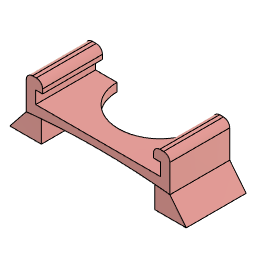
MPR121_Clip (Autodesk Fusion 360 design; units mm, degrees)
Autodesk Fusion 360 part; units mm, degrees
note: some values were not read from the file. Set by a fixed rule: which sketch regions a step uses.
sketch "Clip Sketch" plane through (0, 0, 0) normal (0, 0, 1) x (1, 0, 0)
  line L0 (9.9, 4.75) -> (-9.9, 4.75)
  line L1 (-9.9, 4.75) -> (-9.9, -4.75)
  line L2 (-9.9, -4.75) -> (9.9, -4.75)
  line L3 (9.9, -4.75) -> (9.9, 4.75)
  line L4 (9.9, 4.75) -> (-9.9, -4.75) construction
  line L5 (-9.9, 4.75) -> (9.9, -4.75) construction
  line L6 (-9.9, 4.75) -> (-11.4, 4.75)
  line L7 (-11.4, 4.75) -> (-11.4, -4.75)
  line L8 (-11.4, -4.75) -> (-9.9, -4.75)
  line L9 (-9.9, -4.75) -> (-9.9, 4.75)
  line L10 (9.9, -4.75) -> (11.4, -4.75)
  line L11 (11.4, -4.75) -> (11.4, 4.75)
  line L12 (11.4, 4.75) -> (9.9, 4.75)
  line L13 (9.9, 4.75) -> (9.9, -4.75)
  line L14 (-9.9, -4.75) -> (-8.8, -4.75)
  line L15 (-8.8, -4.75) -> (-8.8, 4.75)
  line L16 (-8.8, 4.75) -> (-9.9, 4.75)
  line L17 (-9.9, 4.75) -> (-9.9, -4.75)
  line L18 (0, 2.5) -> (0, 20)
  line L19 (8.8, -4.75) -> (8.8, 4.75)
  line L20 (9.9, -4.75) -> (8.8, -4.75)
  line L21 (8.8, 4.75) -> (9.9, 4.75)
  line L22 (-11.4, 4.75) -> (-11.4, 0.75)
  dimension "d1" = 19.8
  dimension "d2" = 9.5
  dimension "d3" = 1.5
  dimension "d4" = 1.5
  dimension "d5" = 1.1
  dimension "d18" = 4
  constraint horizontal L0
  constraint perpendicular L0 L1
  constraint parallel L0 L2
  constraint parallel L1 L3
  constraint coincident L4 origin
  constraint coincident L5 origin
  constraint horizontal L6
  constraint vertical L7
  constraint horizontal L8
  constraint vertical L9
  constraint horizontal L10
  constraint vertical L11
  constraint horizontal L12
  constraint vertical L13
  constraint collinear L0 L12
  constraint collinear L2 L8
  constraint horizontal L14
  constraint vertical L15
  constraint horizontal L16
  constraint vertical L17
  constraint coincident L9 L1.end
  constraint symmetric L1.end L18 L2.end
  constraint symmetric L14.end L18 L19.start
  constraint symmetric L15.end L18 L19.end
  constraint symmetric L0.end L18 L0.start
  constraint vertical L22
  constraint coincident L7 L22.end
  constraint collinear L0 L16
  constraint collinear L2 L14
  measures "d1" distance of L1.end L2.end
  measures "d2" distance of L0.end L1.end
  measures "d3" distance of L0.end L6.end
  measures "d4" distance of L2.end L10.end
  measures "d5" distance of L1.end L14.end
  measures "d18" distance of L22.end L6.end
extrude "Extrude1" add sketch "Clip Sketch" along normal blind 2
extrude "Extrude2" add sketch "Clip Sketch" along normal blind 4 contours L3 L10 L11 L12 L13 | L1 L6 L7 L8 L9 L17 L22
extrude "Extrude3" add sketch "Clip Sketch" along normal blind 1.7 from surface at 4 contours L0 L2 L3 L13 L19 L20 L21 | L3 L10 L11 L12 L13 | L0 L1 L2 L9 L14 L15 L16 L17 | L1 L6 L7 L8 L9 L17 L22
fillet "Fillet1" radius 1 4 edges at (11.4, 0, 5.7) (8.8, 0, 5.7) (-8.8, 0, 5.7) (-11.4, 0, 5.7)
extrude "Extrude4" add sketch "Clip Sketch" along normal blind 1.5 contours L1 L6 L7 L8 L9 L17 L22
sketch "Sketch2" plane through (0, 4.75, 0) normal (0, 1, 0) x (-1, 0, 0)
  line L0 (11.4, 0) -> (11.4, 4.7)
  arc A0 (11.4, 4.7) -> (10.4, 5.7) centre (10.4, 4.7) ccw
  line L1 (10.4, 5.7) -> (9.8, 5.7)
  arc A1 (9.8, 5.7) -> (8.8, 4.7) centre (9.8, 4.7) ccw
  line L2 (8.8, 4.7) -> (8.8, 4)
  line L3 (8.8, 4) -> (9.9, 4)
  line L4 (9.9, 4) -> (9.9, 2)
  line L5 (9.9, 2) -> (-9.9, 2)
  line L6 (-9.9, 2) -> (-9.9, 4)
  line L7 (-9.9, 4) -> (-8.8, 4)
  line L8 (-8.8, 4) -> (-8.8, 4.7)
  arc A2 (-8.8, 4.7) -> (-9.8, 5.7) centre (-9.8, 4.7) ccw
  line L9 (-9.8, 5.7) -> (-10.4, 5.7)
  arc A3 (-10.4, 5.7) -> (-11.4, 4.7) centre (-10.4, 4.7) ccw
  line L10 (-11.4, 4.7) -> (-11.4, 0)
  line L11 (-11.4, 0) -> (11.4, 0)
  arc A4 (13.5595, 0) -> (-13.5595, 0) centre (0, -104.625) ccw
  dimension "d24" = 105.5
  dimension "d25" = 13.5595
  dimension "d26" = 13.5595
  constraint coincident L11 A4.start
  constraint coincident L11 A4.end
  measures "d24" radius of A4
  measures "d25" distance of origin A4.start
  measures "d26" distance of origin A4.end
extrude "Extrude5" cut sketch "Sketch2" against normal through all contours L0 L10 L11 A4
sketch "Sketch4" plane through (0, 4.75, 0) normal (0, 1, 0) x (-1, 0, 0)
  arc A0 (11.4, 0.2573) -> (-11.4, 0.2573) centre (0, -104.625) ccw
  line L0 (11.4, 0.2573) -> (11.4, 4.7)
  arc A1 (11.4, 4.7) -> (10.4, 5.7) centre (10.4, 4.7) ccw
  line L1 (10.4, 5.7) -> (9.8, 5.7)
  arc A2 (9.8, 5.7) -> (8.8, 4.7) centre (9.8, 4.7) ccw
  line L2 (8.8, 4.7) -> (8.8, 4)
  line L3 (8.8, 4) -> (9.9, 4)
  line L4 (9.9, 4) -> (9.9, 2)
  line L5 (-9.9, 2) -> (-9.9, 4)
  line L6 (-9.9, 4) -> (-8.8, 4)
  line L7 (-8.8, 4) -> (-8.8, 4.7)
  arc A3 (-8.8, 4.7) -> (-9.8, 5.7) centre (-9.8, 4.7) ccw
  line L8 (-9.8, 5.7) -> (-10.4, 5.7)
  arc A4 (-10.4, 5.7) -> (-11.4, 4.7) centre (-10.4, 4.7) ccw
  line L9 (-11.4, 4.7) -> (-11.4, 0.2573)
  line L10 (-11.4, 0.2573) -> (-14, -3)
  line L11 (-14, -3) -> (-9, -3)
  line L12 (-9, -3) -> (-9, 0.4904)
  line L13 (-11.4, 0.2573) -> (-9, 0.4904)
  line L14 (0, 20) -> (0, 2.5)
  line L15 (11.4, 0.2573) -> (9, 0.4904)
  line L16 (9, -3) -> (9, 0.4904)
  line L17 (14, -3) -> (9, -3)
  line L18 (11.4, 0.2573) -> (14, -3)
  line L19 (9.9, 2) -> (-9.9, 2)
  point P0 (11.4, 0.2573)
  constraint coincident A0.end L9.end
  constraint perpendicular L9 L11
  constraint coincident A0 L12.end
  constraint perpendicular L11 L12
  constraint symmetric A0.end L14 P0
  constraint symmetric L10.end L14 L17.start
  constraint symmetric L11.end L14 L16.start
  constraint symmetric L12.end L14 L15.end
extrude "Extrude7" add sketch "Sketch4" against normal blind 9.5 contours L15 L16 L17 L18 | L10 L11 L12 L13
sketch "Sketch5" plane through (0, 0, 2) normal (0, 0, 1) x (-1, 0, 0)
  line L0 (-9.9, 4.75) -> (-9.9, -4.75)
  line L1 (-9.9, -4.75) -> (9.9, -4.75)
  line L2 (9.9, -4.75) -> (9.9, 4.75)
  line L3 (9.9, 4.75) -> (-9.9, 4.75)
  line L4 (-1.75, 0) -> (-22.5, 0)
  line L5 (-6.5, -4.75) -> (6.5, -4.75)
  line L6 (-6.5, 4.75) -> (6.5, 4.75)
  ellipse E0 centre (0, -4.75) end of major axis (6.5, -4.75) minor radius 6.2609
  line L7 (-6.5, -4.75) -> (6.5, -4.75) construction
  line L8 (0, -11.0109) -> (0, 1.5109) construction
  constraint symmetric L6.start L4 L5.start
  constraint symmetric L6.end L4 L5.end
  constraint coincident L3 L6.start
  constraint coincident L3 L6.end
  constraint coincident E0 L5.start
  constraint coincident E0 L5.end
  constraint coincident E0 L8.start
  constraint coincident E0 L8.end
  constraint midpoint L5 E0.centre
  constraint coincident L5.end L7.end
extrude "Extrude8" cut sketch "Sketch5" against normal through all contours L1 L5 E0 picked at (0.1085, -2.6657)
named bodies: "MPR121 Clip"
